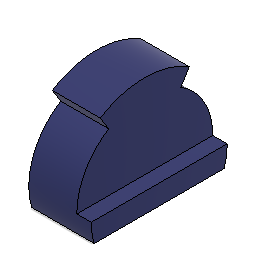
plug-2023.04.23 (Autodesk Fusion 360 design; units mm, degrees)
Autodesk Fusion 360 part; units mm, degrees
sketch "Sketch1" plane through (0, 0, 0) normal (1, 0, 0) x (0, 0, -1)
  circle A0 centre (0, 0) radius 8.5
  line L0 (-9.9073, -2.5) -> (12, -2.5)
  circle A1 centre (0, 0) radius 10.5
  line L1 (-7.5, 12) -> (7.5, 12)
  line L2 (-7.5, 12) -> (0, 0)
  line L3 (0, 0) -> (7.5, 12)
  line L4 (-10.5, -0.0107) -> (10.5, -0.0107)
  point P0 (0, 12)
  dimension "d1" = 17
  dimension "d2" = 2.5
  dimension "d5" = 21
  dimension "d6" = 12
  dimension "d7" = 15
  constraint coincident A0.centre A1.centre
  constraint horizontal L0
  constraint parallel L0 L1
  constraint midpoint L1 P0
  constraint vertical A0.centre P0
  constraint coincident A1 L4.start
  constraint coincident A1 L4.end
  constraint horizontal L4
  measures "d1" diameter of A0
  measures "d2" vertical distance of A0.centre L0.end
  measures "d5" diameter of A1
  measures "d6" distance of A0.centre L1
  measures "d7" distance of L1.start L1.end
extrude "Extrude1" add sketch "Sketch1" along normal blind 6 contours A0 L2 L3 L4 | A0 L2 L3 | A0 A1 L2 L3 | A0 L0 L4
extrude "Extrude2" add sketch "Sketch1" along normal blind 7.8 contours A0 L0 L4
